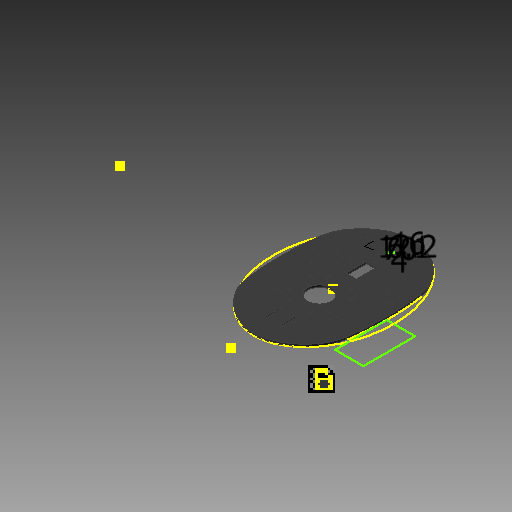
# Autodesk Inventor part: Frame
Saved by Autodesk Inventor 2018 (Build 220112000, 112)
## iProperties
Created: 2017-11-07
Part Number: Frame
Material: Generic
Document SubType Name: Modeling
Designer: kcmat
Density: 1 g/cm^3
Appearance: Default
Author: kcmat
Autodesk Inventor part; units mm, degrees
(part 1 of 2)
ref_plane "YZ Plane" through (0, 0, 0) normal (1, 0, 0) x (0, 1, 0)
ref_plane "XZ Plane" through (0, 0, 0) normal (0, 1, 0) x (-1, 0, 0)
ref_plane "XY Plane" through (0, 0, 0) normal (0, 0, 1) x (1, 0, 0)
sketch "Sketch1" plane through (0, 0, 0) normal (0, 1, 0) x (-1, 0, 0)
  line L0 (0, 0) -> (0, -609.6)
  line L1 (0, -304.8) -> (228.6, -304.8)
  line L2 (0, -304.8) -> (-228.6, -304.8)
  line L3 (228.6, 0) -> (-228.6, 0)
  line L4 (-228.6, 0) -> (-228.6, -609.6)
  line L5 (-228.6, -609.6) -> (228.6, -609.6)
  line L6 (228.6, -609.6) -> (228.6, 0)
  line L7 (0, -304.8) -> (0, -542.544)
  line L8 (0, -542.544) -> (0, -67.056)
  line L9 (0, -304.8) -> (177.8, -304.8)
  line L10 (177.8, -304.8) -> (-177.8, -304.8)
  ellipse E0 centre (0, -304.8) end of major axis (0, -542.544) minor radius 177.8
  dimension "d103" = 237.744
  dimension "d104" = 475.488
  dimension "d105" = 177.8
  dimension "d106" = 355.6
  constraints: 22 end point, 4 point on line, 2 coincident, 2 horizontal, 2 parallel, 2 vertical, 1 midpoint, 1 perpendicular, 4 other
  measures "d103" distance of L2.start L7.end
  measures "d104" distance of L7.end L8.end
  measures "d105" distance of L2.start L9.end
  measures "d106" distance of L9.end L10.end
extrude "Extrusion2" add sketch "Sketch1" along normal blind 6.35 contours E0 L1 L0 | L0 L2 E0 | L1 E0 L0 | L0 E0 L2
sketch "Sketch2" plane through (0, 0, 0) normal (0, -1, 0) x (1, 0, 0)
  line L0 (-18.9386, -143.8342) -> (-18.9385, -150.6384) projected
  arc A0 (-18.9374, -226.1879) -> (-18.9385, -150.6384) centre (-13.97, -188.4131) ccw projected
  line L1 (-18.9374, -226.1879) -> (-18.9373, -233.0223) projected
  arc A1 (-18.9373, -233.0223) -> (-17.829, -230.7308) centre (-21.0349, -230.594) ccw projected
  line L2 (-17.829, -230.7308) -> (-17.7881, -229.5115) projected
  line L3 (-17.7881, -229.5115) -> (-17.788, -229.5111) projected
  arc A2 (-17.788, -229.5111) -> (-15.1337, -229.6717) centre (-13.97, -188.4131) ccw projected
  line L4 (-15.1337, -229.6717) -> (-15.24, -230.8874) projected
  arc A3 (-15.24, -230.8874) -> (-14.2374, -233.4696) centre (-11.4135, -230.8874) ccw projected
  arc A4 (-14.2374, -233.4696) -> (-13.692, -233.4673) centre (-13.97, -232.2276) ccw projected
  arc A5 (-13.692, -233.4673) -> (-12.7, -230.8874) centre (-15.899, -231.138) ccw projected
  line L5 (-12.7, -230.8874) -> (-12.8063, -229.6721) projected
  line L6 (-12.8063, -229.6721) -> (-12.8063, -229.6717) projected
  arc A6 (-12.8063, -229.6717) -> (-10.152, -229.5111) centre (-13.97, -188.4131) ccw projected
  line L7 (-10.152, -229.5111) -> (-10.111, -230.7308) projected
  arc A7 (-10.111, -230.7308) -> (-8.8044, -233.1733) centre (-6.3124, -230.2695) ccw projected
  arc A8 (-8.8044, -233.1733) -> (-8.2633, -233.1053) centre (-8.6887, -231.9082) ccw projected
  arc A9 (-8.2633, -233.1053) -> (-7.5895, -230.4246) centre (-10.735, -231.059) ccw projected
  line L8 (-7.5895, -230.4246) -> (-7.8416, -229.231) projected
  line L9 (-7.8416, -229.231) -> (-7.8417, -229.2306) projected
  arc A10 (-7.8417, -229.2306) -> (-5.226, -228.7512) centre (-13.97, -188.4131) ccw projected
  line L10 (-5.226, -228.7512) -> (-5.0383, -229.9571) projected
  arc A11 (-5.0383, -229.9571) -> (-3.4468, -232.2243) centre (-1.323, -229.0413) ccw projected
  arc A12 (-3.4468, -232.2243) -> (-2.9179, -232.0916) centre (-3.4845, -230.9544) ccw projected
  arc A13 (-2.9179, -232.0916) -> (-2.5721, -229.3492) centre (-5.6182, -230.3581) ccw projected
  line L11 (-2.5721, -229.3492) -> (-2.9662, -228.1947) projected
  line L12 (-2.9662, -228.1947) -> (-2.9663, -228.1943) projected
  arc A14 (-2.9663, -228.1943) -> (-0.4275, -227.4032) centre (-13.97, -188.4131) ccw projected
  line L13 (-0.4275, -227.4032) -> (-0.0959, -228.5776) projected
  arc A15 (-0.0959, -228.5776) -> (1.7573, -230.6365) centre (3.482, -227.2207) ccw projected
  arc A16 (1.7573, -230.6365) -> (2.2664, -230.4409) centre (1.5669, -229.3804) ccw projected
  arc A17 (2.2664, -230.4409) -> (2.2791, -227.6769) centre (-0.6232, -229.0456) ccw projected
  line L14 (2.2791, -227.6769) -> (1.7487, -226.5783) projected
  line L15 (1.7487, -226.5783) -> (1.7485, -226.5779) projected
  arc A18 (1.7485, -226.5779) -> (4.1735, -225.4865) centre (-13.97, -188.4131) ccw projected
  line L16 (4.1735, -225.4865) -> (4.6443, -226.6124) projected
  arc A19 (4.6443, -226.6124) -> (6.7321, -228.4329) centre (8.0325, -224.8341) ccw projected
  arc A20 (6.7321, -228.4329) -> (7.2139, -228.1774) centre (6.3917, -227.2089) ccw projected
  arc A21 (7.2139, -228.1774) -> (6.8933, -225.432) centre (4.1772, -227.1406) ccw projected
  line L17 (6.8933, -225.432) -> (6.2344, -224.4053) projected
  line L18 (6.2344, -224.4053) -> (6.2342, -224.405) projected
  arc A22 (6.2342, -224.405) -> (8.5099, -223.0293) centre (-13.97, -188.4131) ccw projected
  line L19 (8.5099, -223.0293) -> (9.113, -224.0902) projected
  arc A23 (9.113, -224.0902) -> (11.405, -225.6458) centre (12.2621, -221.9165) ccw projected
  arc A24 (11.405, -225.6458) -> (11.8525, -225.3341) centre (10.9195, -224.4717) ccw projected
  arc A25 (11.8525, -225.3341) -> (11.2034, -222.6473) centre (8.713, -224.6708) ccw projected
  line L20 (11.2034, -222.6473) -> (10.4255, -221.7075) projected
  line L21 (10.4255, -221.7075) -> (10.4252, -221.7072) projected
  arc A26 (10.4252, -221.7072) -> (12.5185, -220.0672) centre (-13.97, -188.4131) ccw projected
  line L22 (12.5185, -220.0672) -> (13.2451, -221.0478) projected
  arc A27 (13.2451, -221.0478) -> (15.7079, -222.3157) centre (16.1093, -218.5103) ccw projected
  arc A28 (15.7079, -222.3157) -> (16.1146, -221.9523) centre (15.0844, -221.2087) ccw projected
  arc A29 (16.1146, -221.9523) -> (15.1463, -219.3634) centre (12.918, -221.6723) ccw projected
  line L23 (15.1463, -219.3634) -> (14.2608, -218.5242) projected
  line L24 (14.2608, -218.5242) -> (14.2605, -218.5239) projected
  arc A30 (14.2605, -218.5239) -> (16.1409, -216.6436) centre (-13.97, -188.4131) ccw projected
  line L25 (16.1409, -216.6436) -> (16.9803, -217.5294) projected
  arc A31 (16.9803, -217.5294) -> (19.578, -218.4912) centre (19.5178, -214.6652) ccw projected
  arc A32 (19.578, -218.4912) -> (19.9379, -218.0815) centre (18.8257, -217.4675) ccw projected
  arc A33 (19.9379, -218.0815) -> (18.6647, -215.6281) centre (16.7309, -218.1888) ccw projected
  line L26 (18.6647, -215.6281) -> (17.6844, -214.9018) projected
  line L27 (17.6844, -214.9018) -> (17.6841, -214.9016) projected
  arc A34 (17.6841, -214.9016) -> (19.3241, -212.8083) centre (-13.97, -188.4131) ccw projected
  line L28 (19.3241, -212.8083) -> (20.2643, -213.5864) projected
  arc A35 (20.2643, -213.5864) -> (22.9589, -214.2281) centre (22.4379, -210.4372) ccw projected
  arc A36 (22.9589, -214.2281) -> (23.2668, -213.778) centre (22.0887, -213.3026) ccw projected
  arc A37 (23.2668, -213.778) -> (21.7071, -211.496) centre (20.0961, -214.2711) ccw projected
  line L29 (21.7071, -211.496) -> (20.6465, -210.8932) projected
  line L30 (20.6465, -210.8932) -> (20.6462, -210.893) projected
  arc A38 (20.6462, -210.893) -> (22.0219, -208.6173) centre (-13.97, -188.4131) ccw projected
  line L31 (22.0219, -208.6173) -> (23.049, -209.2764) projected
  arc A39 (23.049, -209.2764) -> (25.8013, -209.5886) centre (24.8272, -205.8882) ccw projected
  arc A40 (25.8013, -209.5886) -> (26.0527, -209.1047) centre (24.8259, -208.7747) ccw projected
  arc A41 (26.0527, -209.1047) -> (24.2293, -207.0273) centre (22.9646, -209.9764) ccw projected
  line L32 (24.2293, -207.0273) -> (23.1038, -206.5567) projected
  line L33 (23.1038, -206.5567) -> (23.1034, -206.5565) projected
  arc A42 (23.1034, -206.5565) -> (24.1948, -204.1316) centre (-13.97, -188.4131) ccw projected
  line L34 (24.1948, -204.1316) -> (25.2939, -204.6622) projected
  arc A43 (25.2939, -204.6622) -> (28.0638, -204.6403) centre (26.6507, -201.0843) ccw projected
  arc A44 (28.0638, -204.6403) -> (28.255, -204.1296) centre (26.9973, -203.9499) ccw projected
  arc A45 (28.255, -204.1296) -> (26.1945, -202.2872) centre (25.2945, -205.3672) ccw projected
  line L35 (26.1945, -202.2872) -> (25.0205, -201.9557) projected
  line L36 (25.0205, -201.9557) -> (25.0201, -201.9555) projected
  arc A46 (25.0201, -201.9555) -> (25.8112, -199.4167) centre (-13.97, -188.4131) ccw projected
  line L37 (25.8112, -199.4167) -> (26.9662, -199.8109) projected
  arc A47 (26.9662, -199.8109) -> (29.7133, -199.4554) centre (27.8819, -196.0956) ccw projected
  arc A48 (29.7133, -199.4554) -> (29.8416, -198.9253) centre (28.5714, -198.8986) ccw projected
  arc A49 (29.8416, -198.9253) -> (27.574, -197.3447) centre (27.0518, -200.5108) ccw projected
  line L38 (27.574, -197.3447) -> (26.3686, -197.1572) projected
  line L39 (26.3686, -197.1572) -> (26.3682, -197.1571) projected
  arc A50 (26.3682, -197.1571) -> (26.8475, -194.5414) centre (-13.97, -188.4131) ccw projected
  line L40 (26.8475, -194.5414) -> (28.0416, -194.7935) projected
  arc A51 (28.0416, -194.7935) -> (30.7258, -194.1094) centre (28.5028, -190.9949) ccw projected
  arc A52 (30.7258, -194.1094) -> (30.7892, -193.5678) centre (29.5251, -193.6943) ccw projected
  arc A53 (30.7892, -193.5678) -> (28.3477, -192.272) centre (28.2109, -195.4779) ccw projected
  line L41 (28.3477, -192.272) -> (27.1284, -192.2311) projected
  line L42 (27.1284, -192.2311) -> (27.128, -192.2311) projected
  arc A54 (27.128, -192.2311) -> (27.2886, -189.5767) centre (-13.97, -188.4131) ccw projected
  line L43 (27.2886, -189.5767) -> (28.5044, -189.6831) projected
  arc A55 (28.5044, -189.6831) -> (31.0866, -188.6804) centre (28.5043, -185.8565) ccw projected
  arc A56 (31.0866, -188.6804) -> (31.0842, -188.1351) centre (29.8446, -188.4131) ccw projected
  arc A57 (31.0842, -188.1351) -> (28.5043, -187.1431) centre (28.7549, -190.3421) ccw projected
  line L44 (28.5043, -187.1431) -> (27.289, -187.2494) projected
  line L45 (27.289, -187.2494) -> (27.2886, -187.2494) projected
  arc A58 (27.2886, -187.2494) -> (27.128, -184.5951) centre (-13.97, -188.4131) ccw projected
  line L46 (27.128, -184.5951) -> (28.3478, -184.5541) projected
  arc A59 (28.3478, -184.5541) -> (30.7903, -183.2475) centre (27.8865, -180.7555) ccw projected
  arc A60 (30.7903, -183.2475) -> (30.7222, -182.7064) centre (29.5251, -183.1318) ccw projected
  arc A61 (30.7222, -182.7064) -> (28.0416, -182.0326) centre (28.6759, -185.1781) ccw projected
  line L47 (28.0416, -182.0326) -> (26.8479, -182.2847) projected
  line L48 (26.8479, -182.2847) -> (26.8475, -182.2847) projected
  arc A62 (26.8475, -182.2847) -> (26.3682, -179.6691) centre (-13.97, -188.4131) ccw projected
  line L49 (26.3682, -179.6691) -> (27.5741, -179.4814) projected
  arc A63 (27.5741, -179.4814) -> (29.8413, -177.8899) centre (26.6583, -175.7661) ccw projected
  arc A64 (29.8413, -177.8899) -> (29.7085, -177.361) centre (28.5714, -177.9275) ccw projected
  arc A65 (29.7085, -177.361) -> (26.9662, -177.0152) centre (27.9751, -180.0613) ccw projected
  line L50 (26.9662, -177.0152) -> (25.8116, -177.4093) projected
  line L51 (25.8116, -177.4093) -> (25.8112, -177.4094) projected
  arc A66 (25.8112, -177.4094) -> (25.0201, -174.8706) centre (-13.97, -188.4131) ccw projected
  line L52 (25.0201, -174.8706) -> (26.1946, -174.5389) projected
  arc A67 (26.1946, -174.5389) -> (28.2534, -172.6858) centre (24.8376, -170.9611) ccw projected
  arc A68 (28.2534, -172.6858) -> (28.0579, -172.1767) centre (26.9973, -172.8762) ccw projected
  arc A69 (28.0579, -172.1767) -> (25.2938, -172.164) centre (26.6625, -175.0662) ccw projected
  line L53 (25.2938, -172.164) -> (24.1952, -172.6944) projected
  line L54 (24.1952, -172.6944) -> (24.1948, -172.6945) projected
  arc A70 (24.1948, -172.6945) -> (23.1034, -170.2696) centre (-13.97, -188.4131) ccw projected
  line L55 (23.1034, -170.2696) -> (24.2294, -169.7988) projected
  arc A71 (24.2294, -169.7988) -> (26.0498, -167.711) centre (22.451, -166.4106) ccw projected
  arc A72 (26.0498, -167.711) -> (25.7943, -167.2292) centre (24.8258, -168.0514) ccw projected
  arc A73 (25.7943, -167.2292) -> (23.0489, -167.5497) centre (24.7575, -170.2658) ccw projected
  line L56 (23.0489, -167.5497) -> (22.0222, -168.2087) projected
  line L57 (22.0222, -168.2087) -> (22.0219, -168.2089) projected
  arc A74 (22.0219, -168.2089) -> (20.6462, -165.9332) centre (-13.97, -188.4131) ccw projected
  line L58 (20.6462, -165.9332) -> (21.7072, -165.3301) projected
  arc A75 (21.7072, -165.3301) -> (23.2627, -163.0381) centre (19.5334, -162.1809) ccw projected
  arc A76 (23.2627, -163.0381) -> (22.951, -162.5906) centre (22.0887, -163.5236) ccw projected
  arc A77 (22.951, -162.5906) -> (20.2642, -163.2397) centre (22.2877, -165.7301) ccw projected
  line L59 (20.2642, -163.2397) -> (19.3245, -164.0176) projected
  line L60 (19.3245, -164.0176) -> (19.3241, -164.0178) projected
  arc A78 (19.3241, -164.0178) -> (17.6841, -161.9246) centre (-13.97, -188.4131) ccw projected
  line L61 (17.6841, -161.9246) -> (18.6647, -161.198) projected
  arc A79 (18.6647, -161.198) -> (19.9326, -158.7352) centre (16.1272, -158.3338) ccw projected
  arc A80 (19.9326, -158.7352) -> (19.5692, -158.3285) centre (18.8256, -159.3586) ccw projected
  arc A81 (19.5692, -158.3285) -> (16.9803, -159.2968) centre (19.2892, -161.5251) ccw projected
  line L62 (16.9803, -159.2968) -> (16.1412, -160.1823) projected
  line L63 (16.1412, -160.1823) -> (16.1409, -160.1826) projected
  arc A82 (16.1409, -160.1826) -> (14.2605, -158.3022) centre (-13.97, -188.4131) ccw projected
  line L64 (14.2605, -158.3022) -> (15.1463, -157.4627) projected
  arc A83 (15.1463, -157.4627) -> (16.1081, -154.865) centre (12.2821, -154.9253) ccw projected
  arc A84 (16.1081, -154.865) -> (15.6984, -154.5052) centre (15.0844, -155.6174) ccw projected
  arc A85 (15.6984, -154.5052) -> (13.2451, -155.7784) centre (15.8057, -157.7122) ccw projected
  line L65 (13.2451, -155.7784) -> (12.5188, -156.7586) projected
  line L66 (12.5188, -156.7586) -> (12.5185, -156.7589) projected
  arc A86 (12.5185, -156.7589) -> (10.4252, -155.1189) centre (-13.97, -188.4131) ccw projected
  line L67 (10.4252, -155.1189) -> (11.2034, -154.1788) projected
  arc A87 (11.2034, -154.1788) -> (11.8451, -151.4841) centre (8.0542, -152.0051) ccw projected
  arc A88 (11.8451, -151.4841) -> (11.3949, -151.1763) centre (10.9195, -152.3544) ccw projected
  arc A89 (11.3949, -151.1763) -> (9.113, -152.7359) centre (11.8881, -154.3469) ccw projected
  line L68 (9.113, -152.7359) -> (8.5101, -153.7966) projected
  line L69 (8.5101, -153.7966) -> (8.5099, -153.7969) projected
  arc A90 (8.5099, -153.7969) -> (6.2342, -152.4212) centre (-13.97, -188.4131) ccw projected
  line L70 (6.2342, -152.4212) -> (6.8933, -151.3941) projected
  arc A91 (6.8933, -151.3941) -> (7.2056, -148.6417) centre (3.5051, -149.6159) ccw projected
  arc A92 (7.2056, -148.6417) -> (6.7216, -148.3903) centre (6.3916, -149.6172) ccw projected
  arc A93 (6.7216, -148.3903) -> (4.6443, -150.2137) centre (7.5933, -151.4785) ccw projected
  line L71 (4.6443, -150.2137) -> (4.1736, -151.3393) projected
  line L72 (4.1736, -151.3393) -> (4.1735, -151.3396) projected
  arc A94 (4.1735, -151.3396) -> (1.7485, -150.2483) centre (-13.97, -188.4131) ccw projected
  line L73 (1.7485, -150.2483) -> (2.2791, -149.1492) projected
  arc A95 (2.2791, -149.1492) -> (2.2573, -146.3793) centre (-1.2988, -147.7923) ccw projected
  arc A96 (2.2573, -146.3793) -> (1.7465, -146.1881) centre (1.5668, -147.4457) ccw projected
  arc A97 (1.7465, -146.1881) -> (-0.0959, -148.2485) centre (2.9841, -149.1486) ccw projected
  line L74 (-0.0959, -148.2485) -> (-0.4274, -149.4226) projected
  line L75 (-0.4274, -149.4226) -> (-0.4275, -149.423) projected
  arc A98 (-0.4275, -149.423) -> (-2.9663, -148.6319) centre (-13.97, -188.4131) ccw projected
  line L76 (-2.9663, -148.6319) -> (-2.5721, -147.4769) projected
  arc A99 (-2.5721, -147.4769) -> (-2.9277, -144.7298) centre (-6.2875, -146.5612) ccw projected
  arc A100 (-2.9277, -144.7298) -> (-3.4577, -144.6015) centre (-3.4845, -145.8717) ccw projected
  arc A101 (-3.4577, -144.6015) -> (-5.0383, -146.869) centre (-1.8723, -147.3913) ccw projected
  line L77 (-5.0383, -146.869) -> (-5.2259, -148.0745) projected
  line L78 (-5.2259, -148.0745) -> (-5.226, -148.0749) projected
  arc A102 (-5.226, -148.0749) -> (-7.8417, -147.5956) centre (-13.97, -188.4131) ccw projected
  line L79 (-7.8417, -147.5956) -> (-7.5895, -146.4015) projected
  arc A103 (-7.5895, -146.4015) -> (-8.2736, -143.7173) centre (-11.3882, -145.9403) ccw projected
  arc A104 (-8.2736, -143.7173) -> (-8.8153, -143.6538) centre (-8.6888, -144.918) ccw projected
  arc A105 (-8.8153, -143.6538) -> (-10.111, -146.0954) centre (-6.9051, -146.2322) ccw projected
  line L80 (-10.111, -146.0954) -> (-10.1519, -147.3146) projected
  line L81 (-10.1519, -147.3146) -> (-10.152, -147.315) projected
  arc A106 (-10.152, -147.315) -> (-12.8063, -147.1545) centre (-13.97, -188.4131) ccw projected
  line L82 (-12.8063, -147.1545) -> (-12.7, -145.9387) projected
  arc A107 (-12.7, -145.9387) -> (-13.7026, -143.3565) centre (-16.5265, -145.9388) ccw projected
  arc A108 (-13.7026, -143.3565) -> (-14.248, -143.3588) centre (-13.97, -144.5985) ccw projected
  arc A109 (-14.248, -143.3588) -> (-15.24, -145.9387) centre (-12.041, -145.6881) ccw projected
  line L83 (-15.24, -145.9387) -> (-15.1337, -147.1541) projected
  line L84 (-15.1337, -147.1541) -> (-15.1337, -147.1545) projected
  arc A110 (-15.1337, -147.1545) -> (-17.788, -147.315) centre (-13.97, -188.4131) ccw projected
  line L85 (-17.788, -147.315) -> (-17.829, -146.0953) projected
  arc A111 (-17.829, -146.0953) -> (-18.9386, -143.8342) centre (-21.6276, -146.5566) ccw projected
  line L86 (-18.9385, -150.6384) -> (-18.9386, -143.8342) projected
  arc A112 (-18.9386, -143.8342) -> (-19.1356, -143.6528) centre (-21.6276, -146.5566) ccw projected
  arc A113 (-19.1356, -143.6528) -> (-19.6767, -143.7209) centre (-19.2513, -144.918) ccw projected
  arc A114 (-19.6767, -143.7209) -> (-20.3505, -146.4015) centre (-17.205, -145.7671) ccw projected
  line L87 (-20.3505, -146.4015) -> (-20.0984, -147.5952) projected
  line L88 (-20.0984, -147.5952) -> (-20.0983, -147.5956) projected
  arc A115 (-20.0983, -147.5956) -> (-22.714, -148.0749) centre (-13.97, -188.4131) ccw projected
  line L89 (-22.714, -148.0749) -> (-22.9017, -146.869) projected
  arc A116 (-22.9017, -146.869) -> (-24.4932, -144.6018) centre (-26.617, -147.7848) ccw projected
  arc A117 (-24.4932, -144.6018) -> (-25.0221, -144.7346) centre (-24.4555, -145.8717) ccw projected
  arc A118 (-25.0221, -144.7346) -> (-25.3679, -147.4769) centre (-22.3218, -146.468) ccw projected
  line L90 (-25.3679, -147.4769) -> (-24.9738, -148.6315) projected
  line L91 (-24.9738, -148.6315) -> (-24.9737, -148.6319) projected
  arc A119 (-24.9737, -148.6319) -> (-27.5125, -149.423) centre (-13.97, -188.4131) ccw projected
  line L92 (-27.5125, -149.423) -> (-27.8441, -148.2485) projected
  arc A120 (-27.8441, -148.2485) -> (-29.6973, -146.1897) centre (-31.422, -149.6055) ccw projected
  arc A121 (-29.6973, -146.1897) -> (-30.2064, -146.3852) centre (-29.5069, -147.4458) ccw projected
  arc A122 (-30.2064, -146.3852) -> (-30.2191, -149.1492) centre (-27.3168, -147.7805) ccw projected
  line L93 (-30.2191, -149.1492) -> (-29.6887, -150.2479) projected
  line L94 (-29.6887, -150.2479) -> (-29.6885, -150.2483) projected
  arc A123 (-29.6885, -150.2483) -> (-32.1135, -151.3396) centre (-13.97, -188.4131) ccw projected
  line L95 (-32.1135, -151.3396) -> (-32.5843, -150.2137) projected
  arc A124 (-32.5843, -150.2137) -> (-34.6721, -148.3932) centre (-35.9725, -151.992) ccw projected
  arc A125 (-34.6721, -148.3932) -> (-35.1539, -148.6487) centre (-34.3317, -149.6172) ccw projected
  arc A126 (-35.1539, -148.6487) -> (-34.8333, -151.3941) centre (-32.1172, -149.6856) ccw projected
  line L96 (-34.8333, -151.3941) -> (-34.1744, -152.4208) projected
  line L97 (-34.1744, -152.4208) -> (-34.1742, -152.4212) projected
  arc A127 (-34.1742, -152.4212) -> (-36.4499, -153.7969) centre (-13.97, -188.4131) ccw projected
  line L98 (-36.4499, -153.7969) -> (-37.053, -152.7359) projected
  arc A128 (-37.053, -152.7359) -> (-39.345, -151.1804) centre (-40.2021, -154.9097) ccw projected
  arc A129 (-39.345, -151.1804) -> (-39.7925, -151.4921) centre (-38.8595, -152.3544) ccw projected
  arc A130 (-39.7925, -151.4921) -> (-39.1434, -154.1788) centre (-36.653, -152.1553) ccw projected
  line L99 (-39.1434, -154.1788) -> (-38.3655, -155.1186) projected
  line L100 (-38.3655, -155.1186) -> (-38.3652, -155.1189) projected
  arc A131 (-38.3652, -155.1189) -> (-40.4585, -156.7589) centre (-13.97, -188.4131) ccw projected
  line L101 (-40.4585, -156.7589) -> (-41.1851, -155.7784) projected
  arc A132 (-41.1851, -155.7784) -> (-43.6479, -154.5105) centre (-44.0493, -158.3159) ccw projected
  arc A133 (-43.6479, -154.5105) -> (-44.0546, -154.8738) centre (-43.0244, -155.6174) ccw projected
  arc A134 (-44.0546, -154.8738) -> (-43.0863, -157.4628) centre (-40.858, -155.1538) ccw projected
  line L102 (-43.0863, -157.4628) -> (-42.2008, -158.3019) projected
  line L103 (-42.2008, -158.3019) -> (-42.2005, -158.3022) projected
  arc A135 (-42.2005, -158.3022) -> (-44.0809, -160.1826) centre (-13.97, -188.4131) ccw projected
  line L104 (-44.0809, -160.1826) -> (-44.9203, -159.2968) projected
  arc A136 (-44.9203, -159.2968) -> (-47.518, -158.3349) centre (-47.4578, -162.161) ccw projected
  arc A137 (-47.518, -158.3349) -> (-47.8779, -158.7447) centre (-46.7657, -159.3587) ccw projected
  arc A138 (-47.8779, -158.7447) -> (-46.6047, -161.198) centre (-44.6709, -158.6373) ccw projected
  line L105 (-46.6047, -161.198) -> (-45.6244, -161.9243) projected
  line L106 (-45.6244, -161.9243) -> (-45.6241, -161.9246) projected
  arc A139 (-45.6241, -161.9246) -> (-47.2641, -164.0179) centre (-13.97, -188.4131) ccw projected
  line L107 (-47.2641, -164.0179) -> (-48.2043, -163.2397) projected
  arc A140 (-48.2043, -163.2397) -> (-50.8989, -162.598) centre (-50.3779, -166.3889) ccw projected
  arc A141 (-50.8989, -162.598) -> (-51.2068, -163.0481) centre (-50.0287, -163.5236) ccw projected
  arc A142 (-51.2068, -163.0481) -> (-49.6471, -165.3301) centre (-48.0361, -162.555) ccw projected
  line L108 (-49.6471, -165.3301) -> (-48.5865, -165.933) projected
  line L109 (-48.5865, -165.933) -> (-48.5862, -165.9332) projected
  arc A143 (-48.5862, -165.9332) -> (-49.9619, -168.2089) centre (-13.97, -188.4131) ccw projected
  line L110 (-49.9619, -168.2089) -> (-50.989, -167.5497) projected
  arc A144 (-50.989, -167.5497) -> (-53.7413, -167.2375) centre (-52.7672, -170.938) ccw projected
  arc A145 (-53.7413, -167.2375) -> (-53.9927, -167.7215) centre (-52.7659, -168.0515) ccw projected
  arc A146 (-53.9927, -167.7215) -> (-52.1693, -169.7988) centre (-50.9046, -166.8498) ccw projected
  line L111 (-52.1693, -169.7988) -> (-51.0438, -170.2694) projected
  line L112 (-51.0438, -170.2694) -> (-51.0434, -170.2696) projected
  arc A147 (-51.0434, -170.2696) -> (-52.1348, -172.6945) centre (-13.97, -188.4131) ccw projected
  line L113 (-52.1348, -172.6945) -> (-53.2339, -172.164) projected
  arc A148 (-53.2339, -172.164) -> (-56.0038, -172.1858) centre (-54.5907, -175.7419) ccw projected
  arc A149 (-56.0038, -172.1858) -> (-56.195, -172.6966) centre (-54.9373, -172.8762) ccw projected
  arc A150 (-56.195, -172.6966) -> (-54.1345, -174.5389) centre (-53.2345, -171.459) ccw projected
  line L114 (-54.1345, -174.5389) -> (-52.9605, -174.8705) projected
  line L115 (-52.9605, -174.8705) -> (-52.9601, -174.8706) projected
  arc A151 (-52.9601, -174.8706) -> (-53.7512, -177.4094) centre (-13.97, -188.4131) ccw projected
  line L116 (-53.7512, -177.4094) -> (-54.9062, -177.0152) projected
  arc A152 (-54.9062, -177.0152) -> (-57.6533, -177.3707) centre (-55.8219, -180.7305) ccw projected
  arc A153 (-57.6533, -177.3707) -> (-57.7816, -177.9008) centre (-56.5114, -177.9276) ccw projected
  arc A154 (-57.7816, -177.9008) -> (-55.514, -179.4814) centre (-54.9918, -176.3154) ccw projected
  line L117 (-55.514, -179.4814) -> (-54.3086, -179.669) projected
  line L118 (-54.3086, -179.669) -> (-54.3082, -179.6691) projected
  arc A155 (-54.3082, -179.6691) -> (-54.7875, -182.2847) centre (-13.97, -188.4131) ccw projected
  line L119 (-54.7875, -182.2847) -> (-55.9816, -182.0326) projected
  arc A156 (-55.9816, -182.0326) -> (-58.6658, -182.7167) centre (-56.4428, -185.8313) ccw projected
  arc A157 (-58.6658, -182.7167) -> (-58.7292, -183.2584) centre (-57.4651, -183.1318) ccw projected
  arc A158 (-58.7292, -183.2584) -> (-56.2877, -184.5541) centre (-56.1509, -181.3482) ccw projected
  line L120 (-56.2877, -184.5541) -> (-55.0684, -184.595) projected
  line L121 (-55.0684, -184.595) -> (-55.068, -184.5951) projected
  arc A159 (-55.068, -184.5951) -> (-55.2286, -187.2494) centre (-13.97, -188.4131) ccw projected
  line L122 (-55.2286, -187.2494) -> (-56.4444, -187.1431) projected
  arc A160 (-56.4444, -187.1431) -> (-59.0266, -188.1457) centre (-56.4443, -190.9696) ccw projected
  arc A161 (-59.0266, -188.1457) -> (-59.0242, -188.6911) centre (-57.7846, -188.4131) ccw projected
  arc A162 (-59.0242, -188.6911) -> (-56.4443, -189.6831) centre (-56.6949, -186.4841) ccw projected
  line L123 (-56.4443, -189.6831) -> (-55.229, -189.5767) projected
  line L124 (-55.229, -189.5767) -> (-55.2286, -189.5767) projected
  arc A163 (-55.2286, -189.5767) -> (-55.068, -192.2311) centre (-13.97, -188.4131) ccw projected
  line L125 (-55.068, -192.2311) -> (-56.2878, -192.272) projected
  arc A164 (-56.2878, -192.272) -> (-58.7303, -193.5786) centre (-55.8265, -196.0707) ccw projected
  arc A165 (-58.7303, -193.5786) -> (-58.6622, -194.1197) centre (-57.4651, -193.6944) ccw projected
  arc A166 (-58.6622, -194.1197) -> (-55.9816, -194.7935) centre (-56.6159, -191.6481) ccw projected
  line L126 (-55.9816, -194.7935) -> (-54.7879, -194.5415) projected
  line L127 (-54.7879, -194.5415) -> (-54.7875, -194.5414) projected
  arc A167 (-54.7875, -194.5414) -> (-54.3082, -197.1571) centre (-13.97, -188.4131) ccw projected
  line L128 (-54.3082, -197.1571) -> (-55.5141, -197.3448) projected
  arc A168 (-55.5141, -197.3448) -> (-57.7813, -198.9362) centre (-54.5983, -201.0601) ccw projected
  arc A169 (-57.7813, -198.9362) -> (-57.6485, -199.4652) centre (-56.5114, -198.8986) ccw projected
  arc A170 (-57.6485, -199.4652) -> (-54.9062, -199.8109) centre (-55.9151, -196.7649) ccw projected
  line L129 (-54.9062, -199.8109) -> (-53.7516, -199.4168) projected
  line L130 (-53.7516, -199.4168) -> (-53.7512, -199.4167) projected
  arc A171 (-53.7512, -199.4167) -> (-52.9601, -201.9555) centre (-13.97, -188.4131) ccw projected
  line L131 (-52.9601, -201.9555) -> (-54.1346, -202.2872) projected
  arc A172 (-54.1346, -202.2872) -> (-56.1934, -204.1404) centre (-52.7776, -205.8651) ccw projected
  arc A173 (-56.1934, -204.1404) -> (-55.9979, -204.6494) centre (-54.9373, -203.9499) ccw projected
  arc A174 (-55.9979, -204.6494) -> (-53.2338, -204.6621) centre (-54.6025, -201.7599) ccw projected
  line L132 (-53.2338, -204.6621) -> (-52.1352, -204.1317) projected
  line L133 (-52.1352, -204.1317) -> (-52.1348, -204.1316) projected
  arc A175 (-52.1348, -204.1316) -> (-51.0434, -206.5565) centre (-13.97, -188.4131) ccw projected
  line L134 (-51.0434, -206.5565) -> (-52.1694, -207.0274) projected
  arc A176 (-52.1694, -207.0274) -> (-53.9898, -209.1152) centre (-50.391, -210.4156) ccw projected
  arc A177 (-53.9898, -209.1152) -> (-53.7343, -209.597) centre (-52.7658, -208.7747) ccw projected
  arc A178 (-53.7343, -209.597) -> (-50.9889, -209.2764) centre (-52.6975, -206.5603) ccw projected
  line L135 (-50.9889, -209.2764) -> (-49.9622, -208.6174) projected
  line L136 (-49.9622, -208.6174) -> (-49.9619, -208.6173) projected
  arc A179 (-49.9619, -208.6173) -> (-48.5862, -210.893) centre (-13.97, -188.4131) ccw projected
  line L137 (-48.5862, -210.893) -> (-49.6472, -211.4961) projected
  arc A180 (-49.6472, -211.4961) -> (-51.2027, -213.7881) centre (-47.4734, -214.6452) ccw projected
  arc A181 (-51.2027, -213.7881) -> (-50.891, -214.2356) centre (-50.0287, -213.3026) ccw projected
  arc A182 (-50.891, -214.2356) -> (-48.2042, -213.5864) centre (-50.2277, -211.0961) ccw projected
  line L138 (-48.2042, -213.5864) -> (-47.2645, -212.8085) projected
  line L139 (-47.2645, -212.8085) -> (-47.2641, -212.8083) projected
  arc A183 (-47.2641, -212.8083) -> (-45.6241, -214.9016) centre (-13.97, -188.4131) ccw projected
  line L140 (-45.6241, -214.9016) -> (-46.6047, -215.6282) projected
  arc A184 (-46.6047, -215.6282) -> (-47.8726, -218.091) centre (-44.0672, -218.4923) ccw projected
  arc A185 (-47.8726, -218.091) -> (-47.5092, -218.4976) centre (-46.7656, -217.4675) ccw projected
  arc A186 (-47.5092, -218.4976) -> (-44.9203, -217.5294) centre (-47.2292, -215.3011) ccw projected
  line L141 (-44.9203, -217.5294) -> (-44.0812, -216.6439) projected
  line L142 (-44.0812, -216.6439) -> (-44.0809, -216.6436) projected
  arc A187 (-44.0809, -216.6436) -> (-42.2005, -218.5239) centre (-13.97, -188.4131) ccw projected
  line L143 (-42.2005, -218.5239) -> (-43.0863, -219.3634) projected
  arc A188 (-43.0863, -219.3634) -> (-44.0481, -221.9611) centre (-40.2221, -221.9008) ccw projected
  arc A189 (-44.0481, -221.9611) -> (-43.6384, -222.321) centre (-43.0244, -221.2087) ccw projected
  arc A190 (-43.6384, -222.321) -> (-41.1851, -221.0477) centre (-43.7457, -219.114) ccw projected
  line L144 (-41.1851, -221.0477) -> (-40.4588, -220.0675) projected
  line L145 (-40.4588, -220.0675) -> (-40.4585, -220.0672) projected
  arc A191 (-40.4585, -220.0672) -> (-38.3652, -221.7072) centre (-13.97, -188.4131) ccw projected
  line L146 (-38.3652, -221.7072) -> (-39.1434, -222.6473) projected
  arc A192 (-39.1434, -222.6473) -> (-39.7851, -225.342) centre (-35.9942, -224.821) ccw projected
  arc A193 (-39.7851, -225.342) -> (-39.3349, -225.6499) centre (-38.8595, -224.4718) ccw projected
  arc A194 (-39.3349, -225.6499) -> (-37.053, -224.0902) centre (-39.8281, -222.4792) ccw projected
  line L147 (-37.053, -224.0902) -> (-36.4501, -223.0296) projected
  line L148 (-36.4501, -223.0296) -> (-36.4499, -223.0293) projected
  arc A195 (-36.4499, -223.0293) -> (-34.1742, -224.405) centre (-13.97, -188.4131) ccw projected
  line L149 (-34.1742, -224.405) -> (-34.8333, -225.432) projected
  arc A196 (-34.8333, -225.432) -> (-35.1456, -228.1844) centre (-31.4451, -227.2103) ccw projected
  arc A197 (-35.1456, -228.1844) -> (-34.6616, -228.4358) centre (-34.3316, -227.2089) ccw projected
  arc A198 (-34.6616, -228.4358) -> (-32.5843, -226.6124) centre (-35.5333, -225.3477) ccw projected
  line L150 (-32.5843, -226.6124) -> (-32.1136, -225.4869) projected
  line L151 (-32.1136, -225.4869) -> (-32.1135, -225.4865) projected
  arc A199 (-32.1135, -225.4865) -> (-29.6885, -226.5779) centre (-13.97, -188.4131) ccw projected
  line L152 (-29.6885, -226.5779) -> (-30.2191, -227.6769) projected
  arc A200 (-30.2191, -227.6769) -> (-30.1973, -230.4469) centre (-26.6412, -229.0338) ccw projected
  arc A201 (-30.1973, -230.4469) -> (-29.6865, -230.6381) centre (-29.5068, -229.3804) ccw projected
  arc A202 (-29.6865, -230.6381) -> (-27.8441, -228.5776) centre (-30.9241, -227.6776) ccw projected
  line L153 (-27.8441, -228.5776) -> (-27.5126, -227.4035) projected
  line L154 (-27.5126, -227.4035) -> (-27.5125, -227.4032) projected
  arc A203 (-27.5125, -227.4032) -> (-24.9737, -228.1943) centre (-13.97, -188.4131) ccw projected
  line L155 (-24.9737, -228.1943) -> (-25.3679, -229.3493) projected
  arc A204 (-25.3679, -229.3493) -> (-25.0123, -232.0964) centre (-21.6525, -230.265) ccw projected
  arc A205 (-25.0123, -232.0964) -> (-24.4823, -232.2246) centre (-24.4555, -230.9545) ccw projected
  arc A206 (-24.4823, -232.2246) -> (-22.9017, -229.9571) centre (-26.0677, -229.4349) ccw projected
  line L156 (-22.9017, -229.9571) -> (-22.7141, -228.7516) projected
  line L157 (-22.7141, -228.7516) -> (-22.714, -228.7512) projected
  arc A207 (-22.714, -228.7512) -> (-20.0983, -229.2306) centre (-13.97, -188.4131) ccw projected
  line L158 (-20.0983, -229.2306) -> (-20.3505, -230.4247) projected
  arc A208 (-20.3505, -230.4247) -> (-19.6664, -233.1089) centre (-16.5518, -230.8858) ccw projected
  arc A209 (-19.6664, -233.1089) -> (-19.1247, -233.1723) centre (-19.2512, -231.9082) ccw projected
  arc A210 (-19.1247, -233.1723) -> (-18.9373, -233.0223) centre (-21.0349, -230.594) ccw projected
  line L159 (-18.9373, -233.0223) -> (-18.9374, -226.1879) projected
  arc A211 (-36.6119, -219.0554) -> (-18.9374, -226.1879) centre (-13.97, -188.4131) ccw projected
  arc A212 (-33.7817, -210.4626) -> (-36.6119, -219.0554) centre (-33.7817, -215.2251) ccw projected
  line L160 (-33.7817, -210.4626) -> (-28.1884, -210.4626) projected
  line L161 (-28.1884, -210.4626) -> (-28.1884, -205.3826) projected
  line L162 (-28.1884, -205.3826) -> (-43.4284, -205.3828) projected
  line L163 (-43.4284, -205.3828) -> (-43.4287, -182.5228) projected
  line L164 (-43.4287, -182.5228) -> (-28.1887, -182.5226) projected
  line L165 (-28.1887, -182.5226) -> (-28.1888, -177.4426) projected
  line L166 (-28.1888, -177.4426) -> (-43.3616, -177.4428) projected
  arc A213 (-47.5604, -170.4327) -> (-43.3616, -177.4428) centre (-43.3616, -172.6803) ccw projected
  arc A214 (-18.9385, -150.6384) -> (-47.5604, -170.4327) centre (-13.97, -188.4131) ccw projected
  line L167 (12.7, -163.1227) -> (-12.7, -163.1227)
  line L168 (12.7, -213.9227) -> (12.7, -163.1227) projected
  line L169 (-12.7, -163.1227) -> (-12.7, -213.9227) projected
  line L170 (12.7, -213.9227) -> (-12.7, -213.9227)
  point P0 (0, 0)
  constraints: 4 end point, 2 horizontal, 2 other
sketch "Sketch3" plane through (0, 0, 0) normal (0, -1, 0) x (1, 0, 0)
  line L0 (-12.7, -163.1227) -> (-12.7, -213.9227)
  line L1 (12.7, -163.1227) -> (-12.7, -163.1227)
  line L2 (12.7, -213.9227) -> (12.7, -163.1227)
  line L3 (12.7, -213.9227) -> (-12.7, -213.9227)
  line L4 (0, -163.1227) -> (0, -158.1227)
  line L5 (0, -213.9227) -> (0, -218.9227)
  line L6 (0.2801, -494.8628) -> (-12.4199, -494.8628)
  line L7 (-12.7, -433.942) -> (0, -433.942)
  line L8 (-12.9801, -357.742) -> (12.4199, -357.742)
  line L9 (12.4199, -418.6628) -> (-12.9801, -418.6628)
  line L10 (0, 0) -> (0, -75)
  line L11 (0, -609.6) -> (0, -396.8872)
  line L12 (12.7, -433.942) -> (-12.7, -433.942)
  line L13 (-12.7, -494.8628) -> (12.7, -494.8628)
  line L14 (0, -433.942) -> (0, -357.742)
  line L15 (-12.9801, -357.742) -> (12.4199, -357.742)
  line L16 (12.4199, -418.6628) -> (-12.9801, -418.6628)
  line L17 (-12.9801, -418.6628) -> (-15.5201, -418.6628)
  line L18 (-15.5201, -418.6628) -> (14.9599, -418.6628)
  line L19 (-15.5201, -418.6628) -> (14.9599, -418.6628)
  line L20 (14.9599, -418.6628) -> (14.9599, -357.742)
  line L21 (14.9599, -357.742) -> (-15.5201, -357.742)
  line L22 (-15.5201, -357.742) -> (-15.5201, -418.6628)
  circle A0 centre (0, -263.5227) radius 35
  point P0 (0.2801, -433.942)
  dimension "d6" = 5
  dimension "d7" = 5
  dimension "d24" = 12.7
  dimension "d25" = 25.4
  dimension "d91" = 75
  dimension "d107" = 76.2
  dimension "d110" = 2.54
  dimension "d111" = 30.48
  dimension "d142" = 70
  constraints: 46 end point, 7 horizontal, 6 parallel, 5 vertical, 3 point on line, 2 coincident, 2 midpoint, 1 centre point, 1 perpendicular, 1 other
  measures "d6" distance of L4.start L4.end
  measures "d7" distance of L5.start L5.end
  measures "d24" distance of L7.start L7.end
  measures "d25" distance of L9.start L9.end
  measures "d91" distance of L10.start L10.end
  measures "d107" distance of L14.start L14.end
  measures "d110" distance of L16.end L17.end
  measures "d111" distance of L17.end L18.end
  measures "d142" diameter of A0
sketch "Sketch9" plane through (0, 0, 0) normal (0, -1, 0) x (1, 0, 0)
  circle A0 centre (18.4114, -134.7953) radius 1.5 projected
  circle A1 centre (18.4168, -127.1453) radius 1.5 projected
  circle A2 centre (-46.3586, -134.7493) radius 1.5 projected
  circle A3 centre (-46.3532, -127.0993) radius 1.5 projected
  circle A4 centre (39.6499, -221.0456) radius 1.5 projected
  circle A5 centre (47.2999, -221.051) radius 1.5 projected
  circle A6 centre (39.6959, -156.2756) radius 1.5 projected
  circle A7 centre (47.3459, -156.281) radius 1.5 projected
  circle A8 centre (-74.853, -220.9642) radius 1.5 projected
  circle A9 centre (-67.203, -220.9697) radius 1.5 projected
  circle A10 centre (-74.807, -156.1942) radius 1.5 projected
  circle A11 centre (-67.157, -156.1997) radius 1.5 projected
  circle A12 centre (18.3301, -249.1855) radius 1.5 projected
  circle A13 centre (18.3355, -241.5355) radius 1.5 projected
  circle A14 centre (-46.4399, -249.1395) radius 1.5 projected
  circle A15 centre (-46.4344, -241.4895) radius 1.5 projected
  line L0 (-32.4258, -209.7492) -> (-32.4258, -207.7492)
  line L1 (-32.4258, -207.7492) -> (-32.4258, -211.7492)
  arc A16 (-30.927, -207.7491) -> (-33.9246, -207.7493) centre (-32.4258, -207.7492) ccw
  arc A17 (-33.9248, -211.7491) -> (-30.9268, -211.7491) centre (-32.4258, -211.7492) ccw
  line L2 (-33.9248, -211.7492) -> (-33.9246, -207.7493)
  line L3 (-30.9268, -211.7491) -> (-30.927, -207.7491)
  arc A18 (-30.927, -200.0992) -> (-33.9246, -200.0993) centre (-32.4258, -200.0993) ccw
  line L4 (-32.4258, -202.0993) -> (-32.4258, -200.0993)
  line L5 (-30.9268, -204.0992) -> (-30.927, -200.0992)
  line L6 (-32.4258, -200.0993) -> (-32.4258, -204.0993)
  line L7 (-33.9248, -204.0992) -> (-33.9246, -200.0993)
  arc A19 (-33.9248, -204.0992) -> (-30.9268, -204.0992) centre (-32.4258, -204.0993) ccw
  arc A20 (33.9251, -200.144) -> (30.9268, -200.0992) centre (32.4256, -200.1453) ccw
  line L8 (32.4256, -202.1453) -> (32.4256, -200.1453)
  line L9 (33.9246, -204.1455) -> (33.9251, -200.144)
  line L10 (32.4256, -200.1453) -> (32.4256, -204.1453)
  line L11 (30.9266, -204.1452) -> (30.9268, -200.0992)
  arc A21 (30.9266, -204.1452) -> (33.9246, -204.1455) centre (32.4256, -204.1453) ccw
  arc A22 (33.919, -207.7521) -> (30.9214, -207.7522) centre (32.4202, -207.7522) ccw
  line L12 (32.4202, -209.7522) -> (32.4202, -207.7522)
  line L13 (33.9192, -211.7521) -> (33.919, -207.7521)
  line L14 (32.4202, -207.7522) -> (32.4202, -211.7522)
  line L15 (30.9212, -211.7521) -> (30.9214, -207.7522)
  arc A23 (30.9212, -211.7521) -> (33.9192, -211.7521) centre (32.4202, -211.7522) ccw
  arc A24 (-30.9319, -314.4894) -> (-33.9295, -314.4894) centre (-32.4307, -314.4895) ccw
  line L16 (-32.4307, -316.4895) -> (-32.4307, -314.4895)
  line L17 (-30.9317, -318.4894) -> (-30.9319, -314.4894)
  line L18 (-32.4307, -314.4895) -> (-32.4307, -318.4895)
  line L19 (-33.9297, -318.4894) -> (-33.9295, -314.4894)
  arc A25 (-33.9297, -318.4894) -> (-30.9317, -318.4894) centre (-32.4307, -318.4895) ccw
  arc A26 (-30.9323, -322.1395) -> (-33.9299, -322.1395) centre (-32.4311, -322.1395) ccw
  line L20 (-32.4311, -324.1395) -> (-32.4311, -322.1395)
  line L21 (-30.9321, -326.1394) -> (-30.9323, -322.1395)
  line L22 (-32.4311, -322.1395) -> (-32.4311, -326.1395)
  line L23 (-33.93, -326.1394) -> (-33.9299, -322.1395)
  arc A27 (-33.93, -326.1394) -> (-30.9321, -326.1394) centre (-32.4311, -326.1395) ccw
  arc A28 (33.8377, -322.1855) -> (30.8401, -322.1854) centre (32.3389, -322.1855) ccw
  line L24 (32.3389, -323.0027) -> (32.3389, -321.0027)
  line L25 (33.8379, -326.1854) -> (33.8377, -322.1855)
  line L26 (32.3389, -322.1855) -> (32.3389, -326.1855)
  line L27 (30.8399, -326.1854) -> (30.8401, -322.1854)
  arc A29 (30.8399, -326.1854) -> (33.8379, -326.1854) centre (32.3389, -326.1855) ccw
  arc A30 (33.8432, -314.5354) -> (30.8456, -314.5355) centre (32.3444, -314.5355) ccw
  line L28 (32.3444, -316.5355) -> (32.3444, -314.5355)
  line L29 (33.8433, -318.5354) -> (33.8432, -314.5354)
  line L30 (32.3444, -314.5355) -> (32.3444, -318.5355)
  line L31 (30.8454, -318.5354) -> (30.8456, -314.5355)
  arc A31 (30.8454, -318.5354) -> (33.8433, -318.5354) centre (32.3444, -318.5355) ccw
  line L32 (-60.8442, -295.9646) -> (-62.8442, -295.9646)
  line L33 (-62.8442, -295.9646) -> (-58.8442, -295.9646)
  arc A32 (-58.8442, -297.4645) -> (-58.8442, -294.4646) centre (-58.8442, -295.9646) ccw
  arc A33 (-62.8442, -294.4646) -> (-62.8442, -297.4645) centre (-62.8442, -295.9646) ccw
  line L34 (-62.8442, -297.4645) -> (-58.8442, -297.4645)
  line L35 (-62.8442, -294.4646) -> (-58.8442, -294.4646)
  line L36 (-53.1942, -295.9642) -> (-55.1942, -295.9642)
  line L37 (-55.1942, -295.9642) -> (-51.1942, -295.9642)
  arc A34 (-51.1942, -297.4641) -> (-51.1942, -294.4643) centre (-51.1942, -295.9642) ccw
  arc A35 (-55.1942, -294.4643) -> (-55.1942, -297.4641) centre (-55.1942, -295.9642) ccw
  line L38 (-55.1942, -297.4641) -> (-51.1942, -297.4641)
  line L39 (-55.1942, -294.4643) -> (-51.1942, -294.4643)
  line L40 (-60.8442, -231.1942) -> (-62.8442, -231.1942)
  line L41 (-62.8442, -231.1942) -> (-58.8442, -231.1942)
  arc A36 (-58.8442, -232.6942) -> (-58.8442, -229.6943) centre (-58.8442, -231.1942) ccw
  arc A37 (-62.8442, -229.6943) -> (-62.8442, -232.6942) centre (-62.8442, -231.1942) ccw
  line L42 (-62.8442, -232.6942) -> (-58.8442, -232.6942)
  line L43 (-62.8442, -229.6943) -> (-58.8442, -229.6943)
  line L44 (-53.1482, -231.1997) -> (-55.1482, -231.1997)
  line L45 (-55.1482, -231.1997) -> (-51.1482, -231.1997)
  arc A38 (-51.1482, -232.6996) -> (-51.1482, -229.6998) centre (-51.1482, -231.1997) ccw
  arc A39 (-55.1482, -229.6998) -> (-55.1482, -232.6996) centre (-55.1482, -231.1997) ccw
  line L46 (-55.1482, -232.6996) -> (-51.1482, -232.6996)
  line L47 (-55.1482, -229.6998) -> (-51.1482, -229.6998)
  line L48 (53.6587, -295.9642) -> (51.6587, -295.9642)
  line L49 (51.6587, -295.9642) -> (55.6587, -295.9642)
  arc A40 (55.6587, -297.4641) -> (55.6587, -294.4643) centre (55.6587, -295.9642) ccw
  arc A41 (51.6587, -294.4643) -> (51.6587, -297.4641) centre (51.6587, -295.9642) ccw
  line L50 (51.6587, -297.4641) -> (55.6587, -297.4641)
  line L51 (51.6587, -294.4643) -> (55.6587, -294.4643)
  line L52 (61.3087, -295.9642) -> (59.3087, -295.9642)
  line L53 (59.3087, -295.9642) -> (63.3087, -295.9642)
  arc A42 (63.3087, -297.4641) -> (63.3087, -294.4643) centre (63.3087, -295.9642) ccw
  arc A43 (59.3087, -294.4643) -> (59.3087, -297.4641) centre (59.3087, -295.9642) ccw
  line L54 (59.3087, -297.4641) -> (63.3087, -297.4641)
  line L55 (59.3087, -294.4643) -> (63.3087, -294.4643)
  line L56 (53.7047, -231.2756) -> (51.7047, -231.2756)
  line L57 (51.7047, -231.2756) -> (55.7047, -231.2756)
  arc A44 (55.7047, -232.7755) -> (55.7047, -229.7757) centre (55.7047, -231.2756) ccw
  arc A45 (51.7047, -229.7757) -> (51.7047, -232.7755) centre (51.7047, -231.2756) ccw
  line L58 (51.7047, -232.7755) -> (55.7047, -232.7755)
  line L59 (51.7047, -229.7757) -> (55.7047, -229.7757)
  line L60 (61.3547, -231.281) -> (59.3547, -231.281)
  line L61 (59.3547, -231.281) -> (63.3547, -231.281)
  arc A46 (63.3547, -232.7809) -> (63.3547, -229.7811) centre (63.3547, -231.281) ccw
  arc A47 (59.3547, -229.7811) -> (59.3547, -232.7809) centre (59.3547, -231.281) ccw
  line L62 (59.3547, -232.7809) -> (63.3547, -232.7809)
  line L63 (59.3547, -229.7811) -> (63.3547, -229.7811)
  line L64 (14.0088, 0) -> (14.0088, -74.9999)
  line L65 (32.3444, -318.5355) -> (32.3389, -322.1855)
  line L66 (-32.4307, -318.4895) -> (-32.4311, -322.1395)
  circle A48 centre (-31.3951, -412.3128) radius 1.25 projected
  circle A49 centre (-21.8701, -415.4878) radius 1.25 projected
  circle A50 centre (-31.3951, -388.1966) radius 1.25 projected
  circle A51 centre (-31.3951, -364.092) radius 1.25 projected
  circle A52 centre (-21.8701, -360.917) radius 1.25 projected
  circle A53 centre (27.1519, -405.5552) radius 1.25 projected
  circle A54 centre (27.1519, -360.7012) radius 1.25 projected
  line L67 (-30.927, -200.0992) -> (30.9268, -200.0992)
  line L68 (14.0088, -200.0992) -> (-16.9182, -200.0992)
  point P0 (0, 0)
  dimension "d48" = 2
  dimension "d49" = 4
  dimension "d58" = 2
  dimension "d59" = 4
  dimension "d60" = 2
  dimension "d61" = 4
  dimension "d62" = 2
  dimension "d63" = 4
  dimension "d64" = 2
  dimension "d65" = 4
  dimension "d66" = 2
  dimension "d67" = 4
  dimension "d68" = 2
  dimension "d69" = 4
  dimension "d70" = 2
  dimension "d71" = 4
  dimension "d73" = 4
  dimension "d74" = 2
  dimension "d75" = 4
  dimension "d76" = 2
  dimension "d77" = 4
  dimension "d78" = 2
  dimension "d79" = 4
  dimension "d80" = 2
  dimension "d81" = 4
  dimension "d82" = 2
  dimension "d83" = 4
  dimension "d84" = 2
  dimension "d85" = 4
  dimension "d86" = 2
  dimension "d87" = 4
  dimension "d90" = 76.297
  dimension "d92" = 3.65
  dimension "d93" = 3.65
  dimension "d141" = 30.927
  constraints: 138 end point, 80 point on circle, 37 coincident, 32 centre point, 25 horizontal, 25 point on line, 16 tangent, 9 vertical
  measures "d48" distance of L0.start L0.end
  measures "d49" distance of L0.end L1.end
  measures "d58" distance of L4.start L4.end
  measures "d59" distance of L4.end L6.end
  measures "d60" distance of L8.start L8.end
  measures "d61" distance of L8.end L10.end
  measures "d62" distance of L12.start L12.end
  measures "d63" distance of L12.end L14.end
  measures "d64" distance of L16.start L16.end
  measures "d65" distance of L16.end L18.end
  measures "d66" distance of L20.start L20.end
  measures "d67" distance of L20.end L22.end
  measures "d68" distance of L24.end L24.start
  measures "d69" distance of L26.start L26.end
  measures "d70" distance of L28.start L28.end
  measures "d71" distance of L28.end L30.end
  measures "d73" distance of L32.end L33.end
  measures "d74" distance of L36.start L36.end
  measures "d75" distance of L36.end L37.end
  measures "d76" distance of L40.start L40.end
  measures "d77" distance of L40.end L41.end
  measures "d78" distance of L44.start L44.end
  measures "d79" distance of L44.end L45.end
  measures "d80" distance of L48.start L48.end
  measures "d81" distance of L48.end L49.end
  measures "d82" distance of L52.start L52.end
  measures "d83" distance of L52.end L53.end
  measures "d84" distance of L56.start L56.end
  measures "d85" distance of L56.end L57.end
  measures "d86" distance of L60.start L60.end
  measures "d87" distance of L60.end L61.end
  measures "d90" distance of point (0, 0) L64.end
  measures "d92" distance of L65.start L65.end
  measures "d93" distance of L66.start L66.end
  measures "d141" distance of L68.start L68.end
extrude "Extrusion13" cut sketch "Sketch9" against normal blind 10 contours L3 A17 L2 A16 | L5 A19 L7 A18 | A20 L9 A21 L11 | L13 A23 L15 A22 | L17 A25 L19 A24 | A26 L21 A27 L23 | L25 A29 L27 A28 | A31 L31 A30 L29 | L34 A33 L35 A32 | L38 A35 L39 A34 | L42 A37 L43 A36 | L46 A39 L47 A38 | L50 A41 L51 A40 | L54 A43 L55 A42 | L58 A45 L59 A44 | L62 A47 L63 A46 | A48 | A49 | A50 | A51 | A52 | A53 | A54
extrude "Extrusion17" cut sketch "Sketch3" against normal blind 10 contours L8 L14 L11 L9 L17 L22 L21 | L8 L21 L20 L18 L9 L11 L14 | A0
sketch "Sketch12" plane through (0, 0, 0) normal (0, -1, 0) x (1, 0, 0)
  ellipse E0 centre (0, -304.8) end of major axis (0, -542.544) minor radius 177.8 projected
  line L0 (0, -542.544) -> (0, -472.544)
  circle A0 centre (0, -473.1677) radius 2
  point P0 (0, 0)
  dimension "d112" = 70
  dimension "d113" = 4
  constraints: 2 end point, 1 centre point, 1 point on line, 1 vertical, 1 vertical alignment, 1 other
  measures "d112" distance of L0.start L0.end
  measures "d113" diameter of A0
sketch "Sketch13" plane through (0, 0, 0) normal (0, -1, 0) x (1, 0, 0)
  circle A0 centre (24.257, -455.2177) radius 1.25 projected
  circle A1 centre (-14.097, -455.2177) radius 1.25 projected
  circle A2 centre (9.275, -529.719) radius 1.25 projected
  circle A3 centre (-9.275, -529.719) radius 1.25 projected
  circle A4 centre (-14.097, -455.2177) radius 1.5
  circle A5 centre (24.257, -455.2177) radius 1.5
  circle A6 centre (17.082, -448.0427) radius 1.25
  circle A7 centre (-6.922, -448.0427) radius 1.25
  circle A8 centre (-6.922, -448.0427) radius 1.5
  circle A9 centre (17.082, -448.0427) radius 1.5
  circle A10 centre (-11.1, -519.544) radius 1.25
  circle A11 centre (-11.1, -511.544) radius 1.25
  circle A12 centre (11.1, -519.544) radius 1.25
  circle A13 centre (11.1, -511.544) radius 1.25
  circle A14 centre (-9.275, -529.719) radius 1.5
  circle A15 centre (9.275, -529.719) radius 1.5
  circle A16 centre (11.1, -519.544) radius 1.5
  circle A17 centre (11.1, -511.544) radius 1.5
  circle A18 centre (-11.1, -519.544) radius 1.5
  circle A19 centre (-11.1, -511.544) radius 1.5
  point P0 (0, 0)
  dimension "d151" = 3
  dimension "d152" = 3
  dimension "d153" = 3
  dimension "d154" = 3
  dimension "d155" = 3
  dimension "d156" = 3
  dimension "d157" = 3
  dimension "d158" = 3
  dimension "d159" = 3
  dimension "d160" = 3
  constraints: 16 centre point, 10 coincident, 12 other
  measures "d151" diameter of A4
  measures "d152" diameter of A5
  measures "d153" diameter of A8
  measures "d154" diameter of A9
  measures "d155" diameter of A14
  measures "d156" diameter of A15
  measures "d157" diameter of A16
  measures "d158" diameter of A17
  measures "d159" diameter of A18
  measures "d160" diameter of A19
extrude "Extrusion19" cut sketch "Sketch13" against normal blind 10 contours A0 | A1 | A2 | A3 | A4 | A5 | A6 | A7 | A8 | A9 | A10 | A11 | A12 | A13 | A14 | A15 | A16 | A17 | A18 | A19
sketch "Sketch14" plane through (0, 0, 0) normal (0, -1, 0) x (1, 0, 0)
  ellipse E0 centre (0, -304.8) end of major axis (0, -542.544) minor radius 177.8 projected
  line L0 (0, -542.544) -> (0, -526.544)
  line L1 (0, -526.544) -> (6.1, -526.544)
  line L2 (6.1, -526.544) -> (-6.1, -526.544)
  line L3 (-6.1, -526.544) -> (6.1, -526.544)
  line L4 (6.1, -526.544) -> (6.1, -519.846)
  line L5 (6.1, -519.846) -> (-6.1, -519.846)
  line L6 (-6.1, -519.846) -> (-6.1, -526.544)
  point P0 (0, 0)
  dimension "d118" = 16
  dimension "d119" = 6.1
  dimension "d120" = 12.2
  constraints: 14 end point, 2 horizontal, 2 parallel, 1 perpendicular, 1 point on line, 1 vertical, 1 vertical alignment, 1 other
  measures "d118" distance of L0.start L0.end
  measures "d119" distance of L0.end L1.end
  measures "d120" distance of L1.end L2.end
sketch "Sketch15" plane through (0, 0, 0) normal (0, -1, 0) x (1, 0, 0)
  circle A0 centre (32.3895, -82.38) radius 1.25
  circle A1 centre (32.3895, -152.23) radius 1.25
  circle A2 centre (-32.3895, -152.23) radius 1.25
  circle A3 centre (-32.3895, -82.38) radius 1.25
  line L0 (0, 0) -> (0, -207.1911)
  line L1 (33.2636, -82.38) -> (-31.5154, -82.38)
  line L2 (32.3895, -152.23) -> (0, -152.23)
  point P0 (0.8741, -152.23)
  point P1 (0, -152.23)
  dimension "d149" = 64.779
  dimension "d150" = 32.3895
  constraints: 6 end point, 4 centre point, 2 horizontal, 1 point on line, 1 vertical
  measures "d149" distance of L1.start L1.end
  measures "d150" distance of L2.start L2.end
extrude "Extrusion21" cut sketch "Sketch15" against normal blind 10
sketch "Sketch16" plane through (0, 0, 0) normal (0, -1, 0) x (1, 0, 0)
  ellipse E0 centre (0, -304.8) end of major axis (0, -542.544) minor radius 177.8 projected
  line L0 (0, -67.056) -> (0, -167.056)
  line L1 (0, -167.056) -> (144.9173, -167.056)
  line L2 (0, -167.056) -> (-144.9173, -167.056)
  line L3 (0, -304.8) -> (56.2239, -304.8)
  line L4 (0, -542.544) -> (0, -442.544)
  line L5 (0, -442.544) -> (144.9173, -442.544)
  line L6 (0, -442.544) -> (-144.9173, -442.544)
  arc A0 (-144.9173, -167.056) -> (-144.9173, -442.544) centre (634.1788, -304.8) ccw
  arc A1 (144.9173, -442.544) -> (144.9173, -167.056) centre (-634.1788, -304.8) ccw
  ellipse E1 centre (0, -304.8) end of major axis (0, -67.056) minor radius 177.8 (144.9173, -442.544) -> (144.9173, -167.056) ccw
  ellipse E2 centre (0, -304.8) end of major axis (0, -67.056) minor radius 177.8 (-144.9173, -167.056) -> (-144.9173, -442.544) ccw
  point P0 (0, 0)
  point P1 (0, -609.6)
  dimension "d125" = 100
  constraints: 14 end point, 6 symmetric about line, 4 point on circle, 3 horizontal, 2 centre point, 1 vertical, 13 other
  measures "d125" distance of L0.start L0.end
extrude "Extrusion22" cut sketch "Sketch16" against normal blind 10 contours A1 E0 | E0 A0
fillet "Fillet1" radius 127 4 edges at (144.9173, 3.175, -442.544) (144.9173, 3.175, -167.056) (-144.9173, 3.175, -442.544) (-144.9173, 3.175, -167.056)
sketch "Sketch17" plane through (0, 0, 0) normal (0, -1, 0) x (1, 0, 0)
  arc A0 (149.2483, -415.2814) -> (149.2483, -194.3186) centre (-634.1788, -304.8) ccw projected
  line L0 (157.0002, -304.8) -> (240.9402, -304.8)
  line L1 (240.9402, -304.8) -> (240.9402, -151.1549)
  line L2 (240.9402, -151.1549) -> (157.0002, -151.1549)
  line L3 (157.0002, -151.1549) -> (157.0002, -304.8)
  point P0 (0, 0)
  constraints: 8 end point, 2 parallel, 1 horizontal, 1 perpendicular, 1 point on circle